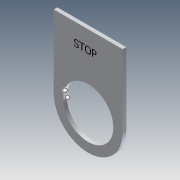
# Autodesk Inventor part: Start Button Lable
Saved by Autodesk Inventor 2016 (Build 200138000, 138)
## iProperties
Created: 2005-06-20
Part Number: Start Button Lable
Checked By: ~
Material: Generic
Document SubType Name: Modeling
Designer: BassBW
Manufacturer: Standard
Standards Organization: Custom
Density: 1 g/cm^3
Appearance: White
SCALE: 1:1
STOCK SIZE: SEE DWG
UNITS: ANSI
COMMODITY: MFG
Author: BassBW
Autodesk Inventor part; units mm, degrees
ref_plane "YZ Plane" through (0, 0, 0) normal (1, 0, 0) x (0, 1, 0)
ref_plane "XZ Plane" through (0, 0, 0) normal (0, 1, 0) x (-1, 0, 0)
ref_plane "XY Plane" through (0, 0, 0) normal (0, 0, 1) x (1, 0, 0)
sketch "Sketch1" plane through (0, 0, 0) normal (0, 0, 1) x (1, 0, 0)
  line L0 (30.1625, 0) -> (30.1625, 31.75)
  line L1 (30.1625, 31.75) -> (0, 31.75)
  line L2 (0, 31.75) -> (0, 0)
  arc A0 (0, 0) -> (30.1625, 0) centre (15.0813, 0) ccw
  dimension "d34" = 30.1625
  dimension "d35" = 31.75
  constraints: 6 end point, 2 point on circle, 2 tangent, 1 centre point, 1 horizontal, 1 parallel, 1 vertical
  measures "d34" distance of L0.end L1.end
  measures "d35" distance from line of A0.centre L1
extrude "Extrusion6" add sketch "Sketch1" along normal blind 1.5875
sketch "Sketch9" plane through (0, 0, 1.5875) normal (0, 0, 1) x (1, 0, 0)
  arc A0 (0, 0) -> (30.1625, 0) centre (15.0813, 0) ccw projected
  circle A1 centre (15.0813, 0) radius 11
  dimension "d38" = 22
  constraints: 1 centre point, 1 coincident
  measures "d38" diameter of A1
extrude "Extrusion7" cut sketch "Sketch9" against normal through all
sketch "Sketch10" plane through (0, 0, 1.5875) normal (0, 0, 1) x (1, 0, 0)
  line L0 (8.7312, 25.4) -> (21.4312, 25.4) construction
  line L1 (21.4312, 25.4) -> (21.4312, 22.225) construction
  line L2 (21.4312, 22.225) -> (8.7312, 22.225) construction
  line L3 (8.7312, 22.225) -> (8.7312, 25.4) construction
  circle A0 centre (15.0813, 0) radius 11 projected
  spline S0 degree 2 poles (9.8897, 22.2334) (9.5587, 22.2334) (9.0943, 22.3718) (8.8893, 22.4706) knots 0 0 0 1 2 2 2
  line L4 (8.8893, 22.4706) -> (8.8893, 22.9794)
  line L5 (8.8893, 22.9794) -> (8.919, 22.9794)
  spline S1 degree 2 poles (8.919, 22.9794) (9.119, 22.7917) (9.6254, 22.5842) (9.86, 22.5842) knots 0 0 0 1 2 2 2
  spline S2 degree 2 poles (9.86, 22.5842) (10.196, 22.5842) (10.5393, 22.8633) (10.5393, 23.093) knots 0 0 0 1 2 2 2
  spline S3 degree 2 poles (10.5393, 23.093) (10.5393, 23.2758) (10.359, 23.503) (10.1639, 23.5598) knots 0 0 0 1 2 2 2
  spline S4 degree 2 poles (10.1639, 23.5598) (10.0231, 23.5994) (9.7884, 23.6537) (9.613, 23.6982) knots 0 0 0 1 2 2 2
  spline S5 degree 2 poles (9.613, 23.6982) (9.455, 23.7401) (9.2055, 23.8661) (9.1092, 23.9674) knots 0 0 0 1 2 2 2
  spline S6 degree 2 poles (9.1092, 23.9674) (9.0153, 24.0687) (8.9116, 24.3404) (8.9116, 24.5182) knots 0 0 0 1 2 2 2
  spline S7 degree 2 poles (8.9116, 24.5182) (8.9116, 24.8887) (9.4895, 25.3901) (9.9366, 25.3901) knots 0 0 0 1 2 2 2
  spline S8 degree 2 poles (9.9366, 25.3901) (10.1935, 25.3901) (10.648, 25.2888) (10.8431, 25.1925) knots 0 0 0 1 2 2 2
  line L6 (10.8431, 25.1925) -> (10.8431, 24.7084)
  line L7 (10.8431, 24.7084) -> (10.8135, 24.7084)
  spline S9 degree 2 poles (10.8135, 24.7084) (10.6677, 24.8418) (10.2133, 25.0394) (9.9638, 25.0394) knots 0 0 0 1 2 2 2
  spline S10 degree 2 poles (9.9638, 25.0394) (9.6822, 25.0394) (9.3339, 24.7751) (9.3339, 24.5602) knots 0 0 0 1 2 2 2
  spline S11 degree 2 poles (9.3339, 24.5602) (9.3339, 24.3675) (9.5389, 24.1378) (9.7316, 24.086) knots 0 0 0 1 2 2 2
  spline S12 degree 2 poles (9.7316, 24.086) (9.86, 24.0514) (10.233, 23.9625) (10.3565, 23.9254) knots 0 0 0 1 2 2 2
  spline S13 degree 2 poles (10.3565, 23.9254) (10.6702, 23.8291) (10.9617, 23.4413) (10.9617, 23.1572) knots 0 0 0 1 2 2 2
  spline S14 degree 2 poles (10.9617, 23.1572) (10.9617, 22.9769) (10.8159, 22.6311) (10.685, 22.5101) knots 0 0 0 1 2 2 2
  spline S15 degree 2 poles (10.685, 22.5101) (10.5393, 22.3767) (10.1688, 22.2334) (9.8897, 22.2334) knots 0 0 0 1 2 2 2
  line L8 (12.0855, 22.2878) -> (12.0855, 24.9752)
  line L9 (12.0855, 24.9752) -> (11.0629, 24.9752)
  line L10 (11.0629, 24.9752) -> (11.0629, 25.3358)
  line L11 (11.0629, 25.3358) -> (13.5132, 25.3358)
  line L12 (13.5132, 25.3358) -> (13.5132, 24.9752)
  line L13 (13.5132, 24.9752) -> (12.4906, 24.9752)
  line L14 (12.4906, 24.9752) -> (12.4906, 22.2878)
  line L15 (12.4906, 22.2878) -> (12.0855, 22.2878)
  spline S16 degree 2 poles (15.9783, 24.9875) (16.1512, 24.785) (16.3438, 24.1922) (16.3438, 23.8118) knots 0 0 0 1 2 2 2
  spline S17 degree 2 poles (16.3438, 23.8118) (16.3438, 23.4413) (16.1561, 22.8411) (15.9783, 22.6385) knots 0 0 0 1 2 2 2
  spline S18 degree 2 poles (15.9783, 22.6385) (15.7906, 22.4261) (15.2941, 22.2236) (14.9952, 22.2236) knots 0 0 0 1 2 2 2
  spline S19 degree 2 poles (14.9952, 22.2236) (14.6865, 22.2236) (14.1925, 22.4335) (14.0121, 22.6385) knots 0 0 0 1 2 2 2
  spline S20 degree 2 poles (14.0121, 22.6385) (13.8368, 22.8411) (13.6491, 23.4363) (13.6491, 23.8118) knots 0 0 0 1 2 2 2
  spline S21 degree 2 poles (13.6491, 23.8118) (13.6491, 24.1946) (13.8392, 24.7776) (14.0146, 24.9875) knots 0 0 0 1 2 2 2
  spline S22 degree 2 poles (14.0146, 24.9875) (14.1925, 25.19) (14.6889, 25.4) (14.9952, 25.4) knots 0 0 0 1 2 2 2
  spline S23 degree 2 poles (14.9952, 25.4) (15.3064, 25.4) (15.8054, 25.1826) (15.9783, 24.9875) knots 0 0 0 1 2 2 2
  spline S24 degree 2 poles (15.9215, 23.8118) (15.9215, 24.1131) (15.7906, 24.58) (15.672, 24.7331) knots 0 0 0 1 2 2 2
  spline S25 degree 2 poles (15.672, 24.7331) (15.551, 24.8912) (15.2101, 25.0493) (14.9977, 25.0493) knots 0 0 0 1 2 2 2
  spline S26 degree 2 poles (14.9977, 25.0493) (14.7778, 25.0493) (14.4469, 24.8961) (14.3209, 24.7331) knots 0 0 0 1 2 2 2
  spline S27 degree 2 poles (14.3209, 24.7331) (14.1999, 24.5775) (14.0714, 24.1082) (14.0714, 23.8118) knots 0 0 0 1 2 2 2
  spline S28 degree 2 poles (14.0714, 23.8118) (14.0714, 23.2116) (14.5753, 22.5743) (14.9977, 22.5743) knots 0 0 0 1 2 2 2
  spline S29 degree 2 poles (14.9977, 22.5743) (15.4201, 22.5743) (15.9215, 23.2116) (15.9215, 23.8118) knots 0 0 0 1 2 2 2
  spline S30 degree 2 poles (18.7151, 24.4169) (18.7151, 24.2193) (18.5743, 23.8636) (18.4483, 23.7401) knots 0 0 0 1 2 2 2
  spline S31 degree 2 poles (18.4483, 23.7401) (18.2902, 23.5845) (17.8629, 23.424) (17.5369, 23.424) knots 0 0 0 1 2 2 2
  line L16 (17.5369, 23.424) -> (17.1935, 23.424)
  line L17 (17.1935, 23.424) -> (17.1935, 22.2878)
  line L18 (17.1935, 22.2878) -> (16.7884, 22.2878)
  line L19 (16.7884, 22.2878) -> (16.7884, 25.3358)
  line L20 (16.7884, 25.3358) -> (17.5541, 25.3358)
  spline S32 degree 2 poles (17.5541, 25.3358) (17.8258, 25.3358) (18.2062, 25.2469) (18.352, 25.1456) knots 0 0 0 1 2 2 2
  spline S33 degree 2 poles (18.352, 25.1456) (18.5224, 25.0295) (18.7151, 24.6713) (18.7151, 24.4169) knots 0 0 0 1 2 2 2
  spline S34 degree 2 poles (18.2927, 24.4046) (18.2927, 24.5627) (18.184, 24.7948) (18.0729, 24.8689) knots 0 0 0 1 2 2 2
  spline S35 degree 2 poles (18.0729, 24.8689) (17.9765, 24.9332) (17.7196, 24.985) (17.5294, 24.985) knots 0 0 0 1 2 2 2
  line L21 (17.5294, 24.985) -> (17.1935, 24.985)
  line L22 (17.1935, 24.985) -> (17.1935, 23.7698)
  line L23 (17.1935, 23.7698) -> (17.4702, 23.7698)
  spline S36 degree 2 poles (17.4702, 23.7698) (17.7172, 23.7698) (18.021, 23.8488) (18.1198, 23.9526) knots 0 0 0 1 2 2 2
  spline S37 degree 2 poles (18.1198, 23.9526) (18.2112, 24.044) (18.2927, 24.2589) (18.2927, 24.4046) knots 0 0 0 1 2 2 2
  dimension "d41" = 3.175
  dimension "d42" = 12.7
  dimension "d43" = 22.225
  dimension "d44" = 6.35
  constraints: 2 other
  measures "d41" distance between parallel lines of L0 L2
  measures "d42" distance between parallel lines of L1 L3
  measures "d43" distance from line of A0.centre L2
  measures "d44" distance from line of A0.centre L3
emboss "Emboss2" sketch "Sketch10" operation cut depth 0.1778 direction (0, 0, -1) contours S0 L4 L5 S1 S2 S3 S4 S5 S6 S7 S8 L6 L7 S9 S10 S11 S12 S13 S14 S15 | L8 L9 L10 L11 L12 L13 L14 L15 | S16 S17 S18 S19 S20 S21 S22 S23 | S30 S31 L16 L17 L18 L19 L20 S32 S33
equation "\"d44\" = 0.5 * d42"
body "Solid1"
